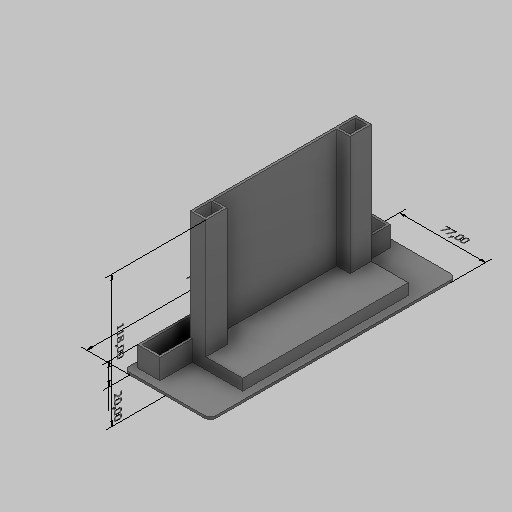
# Autodesk Inventor part: Base do painel vertical
Saved by Autodesk Inventor 2025.2 (Build 292293000, 293)
## iProperties
Created: 2024-05-04
Part Number: Base do painel vertical
Material: Genérico
Document SubType Name: Modeling
Designer: phmca
Density: 1 g/cm^3
Appearance: Padrão
Author: phmca
Autodesk Inventor part; units mm, degrees
ref_plane "YZ Plane" through (0, 0, 0) normal (1, 0, 0) x (0, 1, 0)
ref_plane "XZ Plane" through (0, 0, 0) normal (0, 1, 0) x (-1, 0, 0)
ref_plane "XY Plane" through (0, 0, 0) normal (0, 0, 1) x (1, 0, 0)
sketch "Esboço1" plane through (0, 0, 0) normal (0, 1, 0) x (-1, 0, 0)
  line L0 (-8, 101) -> (8, 101)
  line L1 (8, 101) -> (8, -101)
  line L2 (8, -101) -> (-8, -101)
  line L3 (-8, -101) -> (-8, 101)
  line L4 (-8, 101) -> (8, -101) construction
  line L5 (8, 101) -> (-8, -101) construction
  line L6 (10, 110) -> (-57, 110)
  line L7 (-62, 105) -> (-62, -105)
  line L8 (-57, -110) -> (10, -110)
  line L9 (15, -105) -> (15, 105)
  line L10 (-10, 103) -> (10, 103)
  line L11 (10, 103) -> (10, -103)
  line L12 (10, -103) -> (-10, -103)
  line L13 (-10, -103) -> (-10, 103)
  line L14 (-10, 103) -> (10, -103) construction
  line L15 (10, 103) -> (-10, -103) construction
  line L16 (-10, 74) -> (-55, 74)
  line L17 (-10, -74) -> (-55, -74)
  line L18 (-55, 74) -> (-55, -74)
  arc A0 (15, 105) -> (10, 110) centre (10, 105) ccw
  arc A1 (10, -110) -> (15, -105) centre (10, -105) ccw
  arc A2 (-62, -105) -> (-57, -110) centre (-57, -105) ccw
  arc A3 (-57, 110) -> (-62, 105) centre (-57, 105) ccw
  line L19 (-10, -74) -> (-8, -74)
  line L20 (-10, 74) -> (-8, 74)
  line L21 (-53, 72) -> (-8, 72)
  line L22 (-8, -72) -> (-53, -72)
  line L23 (-53, -72) -> (-53, 72)
  line L24 (-53, 72) -> (-8, -72) construction
  line L25 (-8, 72) -> (-53, -72) construction
  line L26 (-30.5, 0) -> (0, 0) construction
  line L27 (-10, -103) -> (-10, -110) construction
  line L28 (-10, 103) -> (-10, 110) construction
  point P0 (-8, -72)
  dimension "d0" = 16
  dimension "d1" = 202
  dimension "d9" = 7
  dimension "d11" = 2
  dimension "d12" = 2
  dimension "d14" = 45
  dimension "d16" = 45
  dimension "d17" = 5
  dimension "d22" = 2
  dimension "d23" = 2
  dimension "d24" = 2
  dimension "d40" = 220
  dimension "d41" = 7
  dimension "d42" = 7
  dimension "d54" = 148
  constraints: 58 end point, 8 point on circle, 8 point on line, 8 tangent, 7 parallel, 7 perpendicular, 6 horizontal, 6 midpoint, 4 centre point, 3 equal radius, 1 collinear
  measures "d0" distance of L1.end L2.end
  measures "d1" distance of L0.end L1.end
  measures "d9" distance between parallel lines of L9 L1
  measures "d11" distance between parallel lines of L11 L1
  measures "d12" distance between parallel lines of L0 L10
  measures "d14" distance of L16.start L16.end
  measures "d16" distance of L17.start L17.end
  measures "d17" radius of A0
  measures "d22" distance between parallel lines of L17 L22
  measures "d23" distance between parallel lines of L16 L21
  measures "d24" distance between parallel lines of L18 L23
  measures "d40" distance between parallel lines of L6 L8
  measures "d41" distance from line of L16.end L7
  measures "d42" distance between parallel lines of L12 L8
  measures "d54" distance between parallel lines of L16 L17
extrude "Extrusão1" add sketch "Esboço1" along normal blind 2
extrude "Extrusão2" add sketch "Esboço1" along normal blind 20 contours L3 L20 L13 L10 L11 L12 L19 L2 L1 L0
extrude "Extrusão3" add sketch "Esboço1" along normal blind 10 contours L3 L21 L13 L20 | L13 L21 L23 L22 L17 L18 L16 | L3 L19 L13 L22
sketch "Esboço2" plane through (0, 10, 0) normal (0, 1, 0) x (1, 0, 0)
  line L0 (55, -74) -> (55, 74) projected
  line L1 (10, -74) -> (55, -74) projected
  line L2 (10, -74) -> (8, -74) projected
  line L3 (55, 74) -> (10, 74) projected
  line L4 (8, 74) -> (10, 74) projected
  line L5 (53, -72) -> (8, -72) projected
  line L6 (20, -72) -> (20, -57)
  line L7 (20, -57) -> (8, -57)
  line L8 (22, -72) -> (22, -55)
  line L9 (22, -55) -> (8, -55)
  line L10 (8, 101) -> (8, -101) projected
  line L11 (29, 0) -> (13.3569, 0) construction
  line L12 (20, 72) -> (20, 57)
  line L13 (20, 57) -> (8, 57)
  line L14 (22, 72) -> (22, 55)
  line L15 (22, 55) -> (8, 55)
  line L16 (22, -72) -> (22, -74)
  line L17 (20, -72) -> (8, -72)
  line L18 (8, -74) -> (22, -74)
  line L19 (8, -74) -> (8, -72)
  line L20 (22, 72) -> (22, 74)
  line L21 (22, 74) -> (8, 74)
  line L22 (8, 72) -> (53, 72) projected
  line L23 (20, 72) -> (8, 72)
  line L24 (8, 72) -> (8, 74)
  line L25 (8, -55) -> (8, 55)
  line L26 (10, 103) -> (10, -103) projected
  line L27 (10, -55) -> (8, -55)
  line L28 (10, 55) -> (8, 55)
  line L29 (10, -74) -> (10, -74)
  line L30 (10, -74) -> (8, -74)
  line L31 (8, -74) -> (8, -74)
  line L32 (8, -74) -> (10, -74)
  line L33 (10, 74) -> (10, 74)
  line L34 (10, 74) -> (8, 74)
  line L35 (8, 74) -> (8, 74)
  line L36 (10, 74) -> (8, 74)
  point P0 (0, 0)
  point P1 (8, 55)
  point P2 (8, 57)
  dimension "d27" = 2
  dimension "d28" = 2
  dimension "d29" = 12
  dimension "d30" = 15
  dimension "d35" = 0
  dimension "d36" = 0
  constraints: 56 end point, 10 point on line, 7 perpendicular, 6 horizontal, 6 symmetric about line, 6 vertical, 2 collinear, 1 parallel, 5 other
  measures "d27" distance between parallel lines of L9 L7
  measures "d28" distance between parallel lines of L8 L6
  measures "d30" distance between parallel lines of L5 L7
  measures "d35" distance of L1.start L29.end
  measures "d36" distance of L3.end L33.end
extrude "Extrusão4" add sketch "Esboço2" along normal blind 2 contours L1 L16 L8 L9 L26 L15 L14 L20 L3 L0 | L9 L10 L15 L26
extrude "Extrusão5" add sketch "Esboço2" along normal blind 108 contours L1 L26 L5 L16 | L20 L22 L26 L3 | L2 L10 L5 L26 | L5 L6 L7 L26 L9 L8 | L26 L22 L10 L4 | L14 L15 L26 L13 L12 L22 | L7 L10 L9 L26 | L9 L10 L15 L26 | L26 L15 L10 L13
sketch "Esboço4" plane through (0, 0, 0) normal (0, -1, 0) x (1, 0, 0)
  line L0 (-15, -105) -> (-15, 105) projected
  line L1 (-15, 0) -> (62, 0) construction
  line L2 (62, 105) -> (62, -105) projected
  line L3 (23.5, 0) -> (23.5, 110) construction
  line L4 (-10, 110) -> (57, 110) projected
  line L5 (67, -125) -> (-20, -125)
  line L6 (-30, -115) -> (-30, 115)
  line L7 (-20, 125) -> (67, 125)
  line L8 (77, 115) -> (77, -115)
  line L9 (77, -125) -> (-30, 125) construction
  line L10 (-30, -125) -> (77, 125) construction
  arc A0 (-30, -115) -> (-20, -125) centre (-20, -115) ccw
  arc A1 (67, -125) -> (77, -115) centre (67, -115) ccw
  arc A2 (77, 115) -> (67, 125) centre (67, 115) ccw
  arc A3 (-20, 125) -> (-30, 115) centre (-20, 115) ccw
  line L11 (-30, 0) -> (77, 0)
  line L12 (58, -104) -> (-11, -104)
  line L13 (-11, -104) -> (-11, 104)
  line L14 (-11, 104) -> (58, 104)
  line L15 (58, 104) -> (58, -104)
  line L16 (58, -104) -> (-11, 104) construction
  line L17 (-11, -104) -> (58, 104) construction
  line L18 (-8, 101) -> (-8, -101) projected
  line L19 (-8, -101) -> (8, -101) projected
  point P0 (0, 0)
  point P1 (58, 0)
  point P2 (-11, 0)
  dimension "d47" = 10
  dimension "d48" = 3
  dimension "d49" = 3
  dimension "d55" = 15
  dimension "d56" = 15
  constraints: 30 end point, 10 midpoint, 8 point on circle, 8 point on line, 8 tangent, 4 centre point, 4 parallel, 3 equal radius, 2 horizontal, 2 perpendicular
  measures "d47" radius of A0
  measures "d48" distance between parallel lines of L13 L18
  measures "d49" distance between parallel lines of L12 L19
  measures "d55" distance between parallel lines of L7 L4
  measures "d56" distance between parallel lines of L0 L6
extrude "Extrusão6" add sketch "Esboço4" along normal blind 2 separate body contours L5 A0 L6 L11 L13 L12 L15 L8 A1
extrude "Extrusão7" add sketch "Esboço4" along normal blind 2 separate body contours L11 L15 L14 L13 L6 A3 L7 A2 L8
sketch "Esboço5" plane through (0, 118, 0) normal (0, 1, 0) x (1, 0, 0)
  line L0 (8, 72) -> (53, 72) projected
  line L1 (20, 57) -> (8, 57) projected
  line L2 (8, 72) -> (10, 72)
  line L3 (10, 72) -> (10, 57)
  line L4 (10, 57) -> (8, 57)
  line L5 (8, 57) -> (8, 72)
  line L6 (8, -72) -> (8, -101) projected
  line L7 (8, -57) -> (20, -57) projected
  line L8 (8, -72) -> (10, -72)
  line L9 (10, -72) -> (10, -57)
  line L10 (10, -57) -> (8, -57)
  line L11 (8, -57) -> (8, -72)
  point P0 (0, 0)
  point P1 (8, 57)
  dimension "d57" = 2
  dimension "d58" = 2
  constraints: 16 end point, 4 parallel, 2 horizontal, 2 perpendicular, 2 point on line
  measures "d57" distance between parallel lines of L3 L5
  measures "d58" distance between parallel lines of L9 L11
extrude "Extrusão8" add sketch "Esboço5" against normal up to surface (108 mm away) bodies 1
sketch "Esboço6" plane through (0, 12, 0) normal (0, 1, 0) x (1, 0, 0)
  line L0 (10, 55) -> (10, -55) projected
  line L1 (10, -55) -> (22, -55) projected
  line L2 (22, -55) -> (22, -74) projected
  line L3 (22, -74) -> (55, -74) projected
  line L4 (55, -74) -> (55, 74) projected
  line L5 (55, 74) -> (22, 74) projected
  line L6 (22, 74) -> (22, 55) projected
  line L7 (22, 55) -> (10, 55) projected
  line L8 (20, 7.5) -> (12, 7.5)
  line L9 (12, 7.5) -> (12, -7.5)
  line L10 (12, -7.5) -> (20, -7.5)
  line L11 (20, -7.5) -> (20, 7.5)
  line L12 (20, 72) -> (20, 57) projected
  line L13 (10, -9.5) -> (22, -9.5)
  line L14 (22, -9.5) -> (22, 9.5)
  line L15 (22, 9.5) -> (10, 9.5)
  line L16 (10, 9.5) -> (10, -9.5)
  point P0 (0, 0)
  point P1 (10, 0)
  dimension "d69" = 2
  dimension "d70" = 8
  dimension "d71" = 15
  dimension "d72" = 7.5
  dimension "d73" = 2
  dimension "d74" = 2
  dimension "d75" = 2
  dimension "d76" = 2
  constraints: 16 end point, 4 parallel, 2 horizontal, 2 perpendicular, 1 collinear, 1 midpoint, 1 point on line
  measures "d69" distance between parallel lines of L0 L9
  measures "d70" distance of L8.start L8.end
  measures "d71" distance of L10.end L8.start
  measures "d72" distance from line of L10 point (10, 0)
  measures "d73" distance between parallel lines of L16 L9
  measures "d74" distance between parallel lines of L10 L13
  measures "d75" distance between parallel lines of L14 L11
  measures "d76" distance between parallel lines of L15 L8
extrude "Extrusão9" add sketch "Esboço6" along normal blind 35 separate body contours L15 L14 L13 L0
sketch "Esboço7" plane through (10, 12, -55) normal (1, 0, 0) x (0, 0, -1)
  line L0 (0, 0) -> (-110, 0) projected
  line L1 (-72.5, 0) -> (-37.5, 0)
  line L2 (-37.5, 0) -> (-37.5, 2)
  line L3 (-37.5, 2) -> (-72.5, 2)
  line L4 (-72.5, 2) -> (-72.5, 0)
  line L5 (-55, 2) -> (-55, 46.2154)
  line L6 (-64.5, 35) -> (-45.5, 35) projected
  line L7 (-55, 35) -> (-55, 47.2893)
  point P0 (-55, -12)
  dimension "d79" = 35
  dimension "d80" = 2
  constraints: 12 end point, 2 midpoint, 2 parallel, 2 vertical, 1 collinear, 1 horizontal, 1 perpendicular, 1 point on line
  measures "d79" distance of L2.end L3.end
  measures "d80" distance of L3.end L1.start
extrude "Extrusão10" add sketch "Esboço7" along normal blind 20 bodies 4
fillet "Arredondamento1" radius 5 2 edges at (30, 13, 17.5) (30, 13, -17.5)
sketch "Esboço8" plane through (12, 14, -7.5) normal (0, 1, 0) x (1, 0, 0)
  line L0 (0, 0) -> (8, 0) projected
  line L1 (0, -15) -> (0, 0) projected
  line L2 (8, -15) -> (0, -15) projected
  line L3 (8, 0) -> (8, -15) projected
  point P0 (-12, -7.5)
extrude "Extrusão11" cut sketch "Esboço8" against normal up to surface (2 mm away) bodies 4
equation "\"d9\" = d42"
equation "\"d12\" = d11"
equation "\"d16\" = d14"
equation "\"d22\" = d12"
equation "\"d23\" = d22"
equation "\"d24\" = d22"
equation "\"d41\" = d42"
equation "\"d27\" = d28"
equation "\"d72\" = 0.5 * d71"
equation "\"d74\" = d69"
equation "\"d75\" = d69"
equation "\"d76\" = d69"
